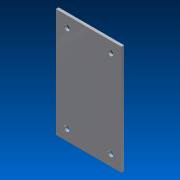
# Autodesk Inventor part: BackSuportPlate
Saved by Autodesk Inventor 2013 (Build 170138000, 138)
## iProperties
Created: 2013-07-23
Part Number: BackSuportPlate
Material: Aluminum 6061
Document SubType Name: Modeling
Designer: orange
Density: 1 g/cm^3
Author: orange
Autodesk Inventor part; units mm, degrees
ref_plane "YZ Plane" through (0, 0, 0) normal (1, 0, 0) x (0, 1, 0)
ref_plane "XZ Plane" through (0, 0, 0) normal (0, 1, 0) x (-1, 0, 0)
ref_plane "XY Plane" through (0, 0, 0) normal (0, 0, 1) x (1, 0, 0)
sketch "Sketch1" plane through (0, 0, 0) normal (0, 0, 1) x (1, 0, 0)
  line L0 (0, 2.1895) -> (76.2, 2.1895)
  line L1 (76.2, 2.1895) -> (76.2, 129.1895)
  line L2 (76.2, 129.1895) -> (0, 129.1895)
  line L3 (0, 129.1895) -> (0, 2.1895)
  point P0 (0, 0)
  dimension "d0" = 127
  dimension "d4" = 76.2
  constraints: 8 end point, 2 parallel, 1 horizontal, 1 perpendicular
  measures "d0" distance of L2.end L0.start
  measures "d4" distance of L0.start L0.end
extrude "Extrusion1" add sketch "Sketch1" along normal blind 3.175
sketch "Sketch2" plane through (0, 0, 3.175) normal (0, 0, 1) x (1, 0, 0)
  line L0 (0, 2.1895) -> (76.2, 2.1895) projected
  line L1 (76.2, 2.1895) -> (76.2, 129.1895) projected
  line L2 (76.2, 129.1895) -> (0, 129.1895) projected
  line L3 (0, 129.1895) -> (0, 2.1895) projected
  point P0 (0, 0)
  point P1 (12.7, 116.4895)
  point P2 (63.5, 116.4895)
  point P3 (12.7, 14.8895)
  point P4 (63.5, 14.8895)
  dimension "d7" = 12.7
  dimension "d8" = 12.7
  dimension "d9" = 12.7
  dimension "d10" = 12.7
  dimension "d11" = 12.7
  dimension "d12" = 12.7
  dimension "d13" = 12.7
  dimension "d14" = 12.7
  measures "d7" distance from line of L0 point (12.7, 14.889)
  measures "d8" distance from line of L3 point (12.7, 14.889)
  measures "d9" distance from line of L2 point (12.7, 116.489)
  measures "d10" distance from line of L3 point (12.7, 116.489)
  measures "d11" distance from line of L2 point (63.5, 116.489)
  measures "d12" distance from line of L1 point (63.5, 116.489)
  measures "d13" distance from line of point (63.5, 14.889) L1
  measures "d14" distance from line of L0 point (63.5, 14.889)
hole "Hole1" at (12.7, 116.4895, 3.175) at (63.5, 116.4895, 3.175) at (12.7, 14.8895, 3.175) at (63.5, 14.8895, 3.175) direction (0, 0, -1) diameter 6.35 end through all
body "Solid1"
